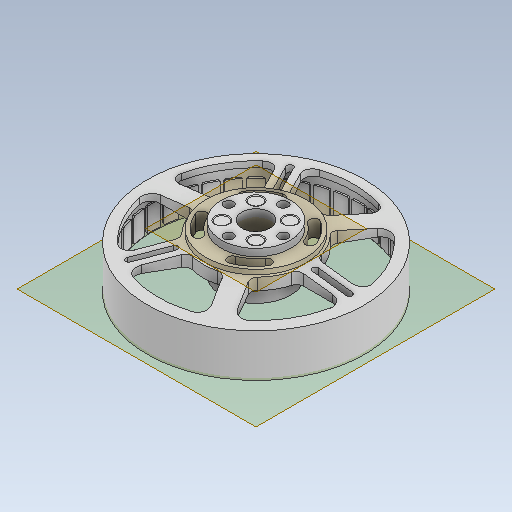
# Autodesk Inventor part: 90motor_top
Saved by Autodesk Inventor 2020 (Build 240168000, 168)
## iProperties
Created: 2020-03-23
Part Number: 90motor_top
Material: Generic
Document SubType Name: Modeling
Designer: psrobotics
Density: 1 g/cm^3
Appearance: Default
Author: psrobotics
Autodesk Inventor part; units mm, degrees
ref_plane "YZ Plane" through (0, 0, 0) normal (1, 0, 0) x (0, 1, 0)
ref_plane "XZ Plane" through (0, 0, 0) normal (0, 1, 0) x (-1, 0, 0)
ref_plane "XY Plane" through (0, 0, 0) normal (0, 0, 1) x (1, 0, 0)
sketch "Sketch1" plane through (0, 0, 0) normal (0, 1, 0) x (-1, 0, 0)
  circle A0 centre (0, 0) radius 45.5
  circle A1 centre (0, 0) radius 43
  dimension "d0" = 91
  dimension "d1" = 2.5
  constraints: 2 centre point, 2 coincident
  measures "d0" diameter of A0
  measures "d1" radial gap between concentric circles of A0 A1
extrude "Extrusion1" add sketch "Sketch1" along normal blind 23
sketch "Sketch2" plane through (0, 23, 0) normal (0, 1, 0) x (1, 0, 0)
  circle A0 centre (0, 0) radius 45.5 projected
extrude "Extrusion2" add sketch "Sketch2" against normal blind 7
sketch "Sketch3" plane through (0, 0, 0) normal (1, 0, 0) x (0, 1, 0)
  line L0 (23, -45.5) -> (23, 45.5) projected
  line L1 (0, -45.5) -> (0, 45.5) projected
  line L2 (23, -45.5) -> (23, 45.5) projected
  line L3 (23, 0) -> (23, -21)
  line L4 (23, -21) -> (21, -21)
  line L5 (0, -45.5) -> (18, -45.5)
  line L6 (0, -45.5) -> (23, -45.5) projected
  line L7 (18, -45.5) -> (21, -21)
  line L8 (23, 0) -> (33, 0)
  point P0 (0, 0)
  dimension "d6" = 21
  dimension "d7" = 2
  dimension "d8" = 18
  dimension "d9" = 10
  constraints: 10 end point, 2 perpendicular, 2 point on line, 1 midpoint
  measures "d6" distance of L3.start L3.end
  measures "d7" distance of L3.end L4.end
  measures "d8" distance of L1.start L5.end
  measures "d9" distance of L3.start L8.end
revolve "Revolution1" cut sketch "Sketch3" angle 360 about axis through (0, 23, 0) along (0, 1, 0)
ref_plane "Work Plane1" through (0, 23, 0) normal (0, 1, 0) x (1, 0, 0)
sketch "Sketch4" plane through (0, 23, 0) normal (0, 1, 0) x (1, 0, 0)
  circle A0 centre (0, 0) radius 21 projected
  circle A1 centre (0, 0) radius 22
  circle A2 centre (0, 0) radius 21 projected
  circle A3 centre (0, 0) radius 41
  line L0 (0, 0) -> (-41, 0)
  line L1 (-22, 0) -> (-41, 0)
  line L2 (-42.5, -4) -> (-42.5, 4)
  line L3 (-42.5, 4) -> (-20.5, 4)
  line L4 (-20.5, 4) -> (-20.5, -4)
  line L5 (-20.5, -4) -> (-42.5, -4)
  line L6 (-42.5, -4) -> (-20.5, 4) construction
  line L7 (-42.5, 4) -> (-20.5, -4) construction
  line L8 (-17.7859, -38.8061) -> (-24.7141, -34.8061)
  line L9 (-24.7141, -34.8061) -> (-13.7141, -15.7535)
  line L10 (-6.7859, -19.7535) -> (-17.7859, -38.8061)
  line L11 (-13.7141, -15.7535) -> (-6.7859, -19.7535)
  line L12 (24.7141, -34.8061) -> (17.7859, -38.8061)
  line L13 (17.7859, -38.8061) -> (6.7859, -19.7535)
  line L14 (13.7141, -15.7535) -> (24.7141, -34.8061)
  line L15 (6.7859, -19.7535) -> (13.7141, -15.7535)
  line L16 (42.5, 4) -> (42.5, -4)
  line L17 (42.5, -4) -> (20.5, -4)
  line L18 (20.5, 4) -> (42.5, 4)
  line L19 (20.5, -4) -> (20.5, 4)
  line L20 (17.7859, 38.8061) -> (24.7141, 34.8061)
  line L21 (24.7141, 34.8061) -> (13.7141, 15.7535)
  line L22 (6.7859, 19.7535) -> (17.7859, 38.8061)
  line L23 (13.7141, 15.7535) -> (6.7859, 19.7535)
  line L24 (-24.7141, 34.8061) -> (-17.7859, 38.8061)
  line L25 (-17.7859, 38.8061) -> (-6.7859, 19.7535)
  line L26 (-13.7141, 15.7535) -> (-24.7141, 34.8061)
  line L27 (-6.7859, 19.7535) -> (-13.7141, 15.7535)
  point P0 (-31.5, 0)
  point P1 (-23.8663, -33.3377)
  point P2 (-14.2808, -16.735)
  point P3 (-21.6333, -4)
  point P4 (-40.8044, -4)
  point P5 (16.9381, -37.3377)
  point P6 (7.3526, -20.735)
  point P7 (-7.3526, -20.735)
  point P8 (-16.9381, -37.3377)
  point P9 (40.8044, -4)
  point P10 (21.6333, -4)
  point P11 (14.2808, -16.735)
  point P12 (23.8663, -33.3377)
  point P13 (23.8663, 33.3377)
  point P14 (14.2808, 16.735)
  point P15 (21.6333, 4)
  point P16 (40.8044, 4)
  point P17 (-16.9381, 37.3377)
  point P18 (-7.3526, 20.735)
  point P19 (7.3526, 20.735)
  point P20 (16.9381, 37.3377)
  point P21 (-14.2808, 16.735)
  point P22 (-23.8663, 33.3377)
  point P23 (-40.8044, 4)
  point P24 (-21.6333, 4)
  dimension "d12" = 44
  dimension "d13" = 82
  dimension "d14" = 8
  dimension "d15" = 22
  dimension "d18" = 360
  constraints: 56 end point, 3 midpoint, 2 coincident, 2 parallel, 2 perpendicular, 1 collinear, 1 horizontal, 1 point on line, 55 other
  measures "d14" distance of L2.start L2.end
  measures "d15" distance of L2.end L3.end
extrude "Extrusion3" cut sketch "Sketch4" against normal blind 7 contours A1 L21 A3 L18 | L17 A3 L14 A1 | A1 L25 A3 L22 | L13 A3 L10 A1 | A1 L3 A3 L26 | L9 A3 L5 A1
fillet "Fillet1" radius 4 2 edges at (-16.9381, 17.2755, 37.3377) (16.9381, 17.2755, 37.3377)
fillet "Fillet2" radius 3 2 edges at (7.3526, 18.4388, 20.735) (-7.3526, 18.4388, 20.735)
pattern_circular "Circular Pattern1" count 6 over 360 about axis through (0, 22, 0) along (0, -1, 0) of "Fillet1", "Fillet2"
sketch "Sketch5" plane through (0, 23, 0) normal (0, 1, 0) x (1, 0, 0)
  line L0 (15.4641, 18.7846) -> (21.5265, 29.285) projected
  arc A0 (40.0302, 8.8649) -> (27.6923, 30.2347) centre (0, 0) ccw projected
  line L1 (36.1248, 4) -> (24, 4) projected
  arc A1 (21.12, 6.16) -> (15.8947, 15.2105) centre (0, 0) ccw projected
  arc A2 (-40.0302, -8.8649) -> (-27.6923, -30.2347) centre (0, 0) ccw projected
  line L2 (-36.1248, -4) -> (-24, -4) projected
  arc A3 (-21.12, -6.16) -> (-15.8947, -15.2105) centre (0, 0) ccw projected
  line L3 (-15.4641, -18.7846) -> (-21.5265, -29.285) projected
  arc A4 (12.3379, 39.0996) -> (-12.3379, 39.0996) centre (0, 0) ccw projected
  line L4 (14.5983, 33.285) -> (8.5359, 22.7846) projected
  arc A5 (5.2253, 21.3705) -> (-5.2253, 21.3705) centre (0, 0) ccw projected
  line L5 (-8.5359, 22.7846) -> (-14.5983, 33.285) projected
  line L6 (21.5265, -29.285) -> (15.4641, -18.7846) projected
  arc A6 (15.8947, -15.2105) -> (21.12, -6.16) centre (0, 0) ccw projected
  line L7 (24, -4) -> (36.1248, -4) projected
  arc A7 (27.6923, -30.2347) -> (40.0302, -8.8649) centre (0, 0) ccw projected
  line L8 (-14.5983, -33.285) -> (-8.5359, -22.7846) projected
  arc A8 (-5.2253, -21.3705) -> (5.2253, -21.3705) centre (0, 0) ccw projected
  line L9 (8.5359, -22.7846) -> (14.5983, -33.285) projected
  arc A9 (-12.3379, -39.0996) -> (12.3379, -39.0996) centre (0, 0) ccw projected
  arc A10 (-15.8947, 15.2105) -> (-21.12, 6.16) centre (0, 0) ccw projected
  line L10 (-24, 4) -> (-36.1248, 4) projected
  arc A11 (-27.6923, 30.2347) -> (-40.0302, 8.8649) centre (0, 0) ccw projected
  line L11 (-21.5265, 29.285) -> (-15.4641, 18.7846) projected
  circle A12 centre (0, 0) radius 45.5 projected
  circle A13 centre (0, 0) radius 21 projected
  line L12 (0, 0) -> (-22.75, -39.4042)
  line L13 (-10.5, -18.1865) -> (-21.5, -37.2391)
  line L14 (-19.5, -33.775) -> (-12.5, -21.6506) construction
  line L15 (-18.4175, -34.4) -> (-11.4175, -22.2756)
  line L16 (-13.5825, -21.0256) -> (-20.5825, -33.15)
  arc A14 (-20.5825, -33.15) -> (-18.4175, -34.4) centre (-19.5, -33.775) ccw
  arc A15 (-11.4175, -22.2756) -> (-13.5825, -21.0256) centre (-12.5, -21.6506) ccw
  point P0 (-16, -27.7128)
  dimension "d27" = 22
  dimension "d28" = 7
  dimension "d29" = 2.5
  constraints: 12 end point, 4 point on circle, 4 tangent, 3 point on line, 2 centre point, 2 midpoint, 2 parallel, 28 other
  measures "d27" distance of L13.start L13.end
  measures "d28" distance of point (-16, -27.713) L14.end
  measures "d29" diameter of A15
extrude "Extrusion4" cut sketch "Sketch5" against normal blind 7 contours A15 L15 A14 L12 | L12 A14 L16 A15
pattern_circular "Circular Pattern2" count 3 over 360 about axis through (0, 23, 0) along (0, -1, 0) of "Extrusion4"
sketch "Sketch6" plane through (0, 23, 0) normal (0, 1, 0) x (1, 0, 0)
  circle A0 centre (0, 0) radius 21 projected
  circle A1 centre (0, 0) radius 14.5
  dimension "d35" = 29
  constraints: 1 centre point, 1 coincident
  measures "d35" diameter of A1
extrude "Extrusion5" add sketch "Sketch6" along normal blind 3 contours A1
sketch "Sketch7" plane through (0, 26, 0) normal (0, 1, 0) x (1, 0, 0)
  circle A0 centre (0, 0) radius 14.5 projected
  line L0 (0, 0) -> (0, -11.45)
  circle A1 centre (0, -11.45) radius 2
  dimension "d38" = 11.45
  dimension "d39" = 4
  constraints: 2 end point, 1 centre point, 1 coincident, 1 vertical
  measures "d38" distance of L0.start L0.end
  measures "d39" diameter of A1
extrude "Extrusion6" cut sketch "Sketch7" against normal blind 20 contours A1
pattern_circular "Circular Pattern3" count 4 over 360 about axis through (0, 23, 0) along (0, 1, 0) of "Extrusion6"
sketch "Sketch8" plane through (0, 26, 0) normal (0, 1, 0) x (1, 0, 0)
  circle A0 centre (0, 0) radius 5.9
  dimension "d45" = 11.8
  constraints: 1 centre point, 1 coincident
  measures "d45" diameter of A0
extrude "Extrusion7" cut sketch "Sketch8" against normal blind 20
sketch "Sketch9" plane through (0, 16, 0) normal (0, -1, 0) x (1, 0, 0)
  circle A0 centre (0, 0) radius 14.5 projected
  circle A1 centre (0, 0) radius 5.9 projected
  circle A2 centre (-11.45, 0) radius 2 projected
  circle A3 centre (0, -11.45) radius 2 projected
  circle A4 centre (11.45, 0) radius 2 projected
  circle A5 centre (0, 11.45) radius 2 projected
  arc A6 (25, 1.25) -> (25, -1.25) centre (25, 0) ccw projected
  line L0 (25, 1.25) -> (39, 1.25) projected
  arc A7 (39, -1.25) -> (39, 1.25) centre (39, 0) ccw projected
  line L1 (39, -1.25) -> (25, -1.25) projected
  arc A8 (-11.4175, -22.2756) -> (-13.5825, -21.0256) centre (-12.5, -21.6506) ccw projected
  line L2 (-11.4175, -22.2756) -> (-18.4175, -34.4) projected
  arc A9 (-20.5825, -33.15) -> (-18.4175, -34.4) centre (-19.5, -33.775) ccw projected
  line L3 (-20.5825, -33.15) -> (-13.5825, -21.0256) projected
  arc A10 (-13.5825, 21.0256) -> (-11.4175, 22.2756) centre (-12.5, 21.6506) ccw projected
  line L4 (-13.5825, 21.0256) -> (-20.5825, 33.15) projected
  arc A11 (-18.4175, 34.4) -> (-20.5825, 33.15) centre (-19.5, 33.775) ccw projected
  line L5 (-18.4175, 34.4) -> (-11.4175, 22.2756) projected
  line L6 (21.5265, -29.285) -> (15.4641, -18.7846) projected
  arc A12 (15.8947, -15.2105) -> (15.4641, -18.7846) centre (18.0622, -17.2846) ccw projected
  arc A13 (15.8947, -15.2105) -> (21.12, -6.16) centre (0, 0) ccw projected
  arc A14 (24, -4) -> (21.12, -6.16) centre (24, -7) ccw projected
  line L7 (24, -4) -> (36.1248, -4) projected
  arc A15 (40.0302, -8.8649) -> (36.1248, -4) centre (36.1248, -8) ccw projected
  arc A16 (27.6923, -30.2347) -> (40.0302, -8.8649) centre (0, 0) ccw projected
  arc A17 (21.5265, -29.285) -> (27.6923, -30.2347) centre (24.9906, -27.285) ccw projected
  arc A18 (-27.6923, 30.2347) -> (-40.0302, 8.8649) centre (0, 0) ccw projected
  arc A19 (-21.5265, 29.285) -> (-27.6923, 30.2347) centre (-24.9906, 27.285) ccw projected
  line L8 (-21.5265, 29.285) -> (-15.4641, 18.7846) projected
  arc A20 (-15.8947, 15.2105) -> (-15.4641, 18.7846) centre (-18.0622, 17.2846) ccw projected
  arc A21 (-15.8947, 15.2105) -> (-21.12, 6.16) centre (0, 0) ccw projected
  arc A22 (-24, 4) -> (-21.12, 6.16) centre (-24, 7) ccw projected
  line L9 (-24, 4) -> (-36.1248, 4) projected
  arc A23 (-40.0302, 8.8649) -> (-36.1248, 4) centre (-36.1248, 8) ccw projected
  arc A24 (-12.3379, -39.0996) -> (12.3379, -39.0996) centre (0, 0) ccw projected
  arc A25 (-14.5983, -33.285) -> (-12.3379, -39.0996) centre (-11.1342, -35.285) ccw projected
  line L10 (-14.5983, -33.285) -> (-8.5359, -22.7846) projected
  arc A26 (-5.2253, -21.3705) -> (-8.5359, -22.7846) centre (-5.9378, -24.2846) ccw projected
  arc A27 (-5.2253, -21.3705) -> (5.2253, -21.3705) centre (0, 0) ccw projected
  arc A28 (8.5359, -22.7846) -> (5.2253, -21.3705) centre (5.9378, -24.2846) ccw projected
  line L11 (8.5359, -22.7846) -> (14.5983, -33.285) projected
  arc A29 (12.3379, -39.0996) -> (14.5983, -33.285) centre (11.1342, -35.285) ccw projected
  line L12 (15.4641, 18.7846) -> (21.5265, 29.285) projected
  arc A30 (27.6923, 30.2347) -> (21.5265, 29.285) centre (24.9906, 27.285) ccw projected
  arc A31 (40.0302, 8.8649) -> (27.6923, 30.2347) centre (0, 0) ccw projected
  arc A32 (36.1248, 4) -> (40.0302, 8.8649) centre (36.1248, 8) ccw projected
  line L13 (36.1248, 4) -> (24, 4) projected
  arc A33 (21.12, 6.16) -> (24, 4) centre (24, 7) ccw projected
  arc A34 (21.12, 6.16) -> (15.8947, 15.2105) centre (0, 0) ccw projected
  arc A35 (15.4641, 18.7846) -> (15.8947, 15.2105) centre (18.0622, 17.2846) ccw projected
  line L14 (-8.5359, 22.7846) -> (-14.5983, 33.285) projected
  arc A36 (-12.3379, 39.0996) -> (-14.5983, 33.285) centre (-11.1342, 35.285) ccw projected
  arc A37 (12.3379, 39.0996) -> (-12.3379, 39.0996) centre (0, 0) ccw projected
  arc A38 (14.5983, 33.285) -> (12.3379, 39.0996) centre (11.1342, 35.285) ccw projected
  line L15 (14.5983, 33.285) -> (8.5359, 22.7846) projected
  arc A39 (5.2253, 21.3705) -> (8.5359, 22.7846) centre (5.9378, 24.2846) ccw projected
  arc A40 (5.2253, 21.3705) -> (-5.2253, 21.3705) centre (0, 0) ccw projected
  arc A41 (-8.5359, 22.7846) -> (-5.2253, 21.3705) centre (-5.9378, 24.2846) ccw projected
  arc A42 (-21.12, -6.16) -> (-15.8947, -15.2105) centre (0, 0) ccw projected
  arc A43 (-15.4641, -18.7846) -> (-15.8947, -15.2105) centre (-18.0622, -17.2846) ccw projected
  line L16 (-15.4641, -18.7846) -> (-21.5265, -29.285) projected
  arc A44 (-27.6923, -30.2347) -> (-21.5265, -29.285) centre (-24.9906, -27.285) ccw projected
  arc A45 (-40.0302, -8.8649) -> (-27.6923, -30.2347) centre (0, 0) ccw projected
  arc A46 (-36.1248, -4) -> (-40.0302, -8.8649) centre (-36.1248, -8) ccw projected
  line L17 (-36.1248, -4) -> (-24, -4) projected
  arc A47 (-21.12, -6.16) -> (-24, -4) centre (-24, -7) ccw projected
  circle A48 centre (0, 0) radius 43 projected
extrude "Extrusion8" add sketch "Sketch9" along normal blind 10 contours A0
sketch "Sketch10" plane through (0, 23, 0) normal (0, 1, 0) x (1, 0, 0)
  circle A0 centre (0, 0) radius 14.5 projected
  circle A1 centre (0, 0) radius 21 projected
  circle A2 centre (0, 0) radius 19.5
  circle A3 centre (0, 0) radius 15.5
  line L0 (0, 0) -> (0, 19.5)
  line L1 (0, 0) -> (-19.5, 0)
  line L2 (0, 0) -> (-5.047, 18.8356)
  line L3 (0, 0) -> (-17.2175, 9.1547)
  point P0 (-13.6857, 7.2768)
  point P1 (-4.0117, 14.9719)
  dimension "d50" = 39
  dimension "d51" = 31
  dimension "d52" = 15
  dimension "d53" = 28
  constraints: 8 end point, 4 point on circle, 2 centre point, 2 coincident, 1 perpendicular, 1 vertical
  measures "d50" diameter of A2
  measures "d51" diameter of A3
  measures "d52" angle of L0 L2
  measures "d53" angle of L1 L3
extrude "Extrusion9" cut sketch "Sketch10" against normal blind 10 contours A3 L3 A2 L2
fillet "Fillet3" radius 2 4 edges at (-17.2175, 19.5, -9.1547) (-13.6857, 19.5, -7.2768) (-4.0117, 19.5, -14.9719) (-5.047, 19.5, -18.8356)
pattern_circular "Circular Pattern4" count 4 over 360 about axis through (0, 26, 0) along (0, -1, 0) of "Extrusion9", "Fillet3"
sketch "Sketch11" plane through (0, 26, 0) normal (0, 1, 0) x (1, 0, 0)
  circle A0 centre (0, 0) radius 5.9 projected
  circle A1 centre (-11.45, 0) radius 2 projected
  circle A2 centre (0, 11.45) radius 2 projected
  circle A3 centre (11.45, 0) radius 2 projected
  circle A4 centre (0, -11.45) radius 2 projected
  circle A5 centre (0, 0) radius 14.5 projected
  line L0 (0, 11.45) -> (11.45, 0)
  line L1 (5.725, 5.725) -> (7.1392, 7.1392)
  circle A6 centre (7.1392, 7.1392) radius 3
  dimension "d60" = 2
  dimension "d61" = 6
  constraints: 4 end point, 1 centre point, 1 coincident, 1 midpoint, 1 perpendicular
  measures "d60" distance of L1.start L1.end
  measures "d61" diameter of A6
extrude "Extrusion10" cut sketch "Sketch11" against normal blind 0.2 contours A6 L0 | L0 A6
pattern_circular "Circular Pattern5" count 4 over 360 about axis through (0, 23, 0) along (0, 1, 0) of "Extrusion10"
fillet "Fillet4" radius 0.5 4 edges at (-7.1392, 25.8, -4.1392) (4.1392, 25.8, -7.1392) (7.1392, 25.8, 4.1392) (-4.1392, 25.8, 7.1392)
thicken "Thicken1" operation add thickness 0.5 both sides no extend neighbours yes toward (-0.8829476, 0, 0.4694716) faces at (-37.9667, 10.6667, 20.1873)
ref_plane "Work Plane2" through (0, 1, 0) normal (0, -1, 0) x (1, 0, 0)
sketch "Sketch12" plane through (0, 1, 0) normal (0, -1, 0) x (1, 0, 0)
  circle A0 centre (0, 0) radius 43.5 projected
  arc A1 (-8.7932, 12.7644) -> (-14.4153, 5.6965) centre (0, 0) ccw projected
  arc A2 (-18.1353, 7.1665) -> (-14.4153, 5.6965) centre (-16.2753, 6.4315) ccw projected
  arc A3 (-11.0624, 16.0584) -> (-18.1353, 7.1665) centre (0, 0) ccw projected
  arc A4 (-8.7932, 12.7644) -> (-11.0624, 16.0584) centre (-9.9278, 14.4114) ccw projected
  arc A5 (12.7644, 8.7932) -> (5.6965, 14.4153) centre (0, 0) ccw projected
  arc A6 (7.1665, 18.1353) -> (5.6965, 14.4153) centre (6.4315, 16.2753) ccw projected
  arc A7 (16.0584, 11.0624) -> (7.1665, 18.1353) centre (0, 0) ccw projected
  arc A8 (12.7644, 8.7932) -> (16.0584, 11.0624) centre (14.4114, 9.9278) ccw projected
  arc A9 (8.7932, -12.7644) -> (14.4153, -5.6965) centre (0, 0) ccw projected
  arc A10 (18.1353, -7.1665) -> (14.4153, -5.6965) centre (16.2753, -6.4315) ccw projected
  arc A11 (11.0624, -16.0584) -> (18.1353, -7.1665) centre (0, 0) ccw projected
  arc A12 (8.7932, -12.7644) -> (11.0624, -16.0584) centre (9.9278, -14.4114) ccw projected
  arc A13 (-12.7644, -8.7932) -> (-5.6965, -14.4153) centre (0, 0) ccw projected
  arc A14 (-7.1665, -18.1353) -> (-5.6965, -14.4153) centre (-6.4315, -16.2753) ccw projected
  arc A15 (-16.0584, -11.0624) -> (-7.1665, -18.1353) centre (0, 0) ccw projected
  arc A16 (-12.7644, -8.7932) -> (-16.0584, -11.0624) centre (-14.4114, -9.9278) ccw projected
  circle A17 centre (0, 0) radius 14.5 projected
  arc A18 (25, 1.25) -> (25, -1.25) centre (25, 0) ccw projected
  line L0 (25, 1.25) -> (39, 1.25) projected
  arc A19 (39, -1.25) -> (39, 1.25) centre (39, 0) ccw projected
  line L1 (39, -1.25) -> (25, -1.25) projected
  arc A20 (-11.4175, -22.2756) -> (-13.5825, -21.0256) centre (-12.5, -21.6506) ccw projected
  line L2 (-11.4175, -22.2756) -> (-18.4175, -34.4) projected
  arc A21 (-20.5825, -33.15) -> (-18.4175, -34.4) centre (-19.5, -33.775) ccw projected
  line L3 (-20.5825, -33.15) -> (-13.5825, -21.0256) projected
  arc A22 (-13.5825, 21.0256) -> (-11.4175, 22.2756) centre (-12.5, 21.6506) ccw projected
  line L4 (-13.5825, 21.0256) -> (-20.5825, 33.15) projected
  arc A23 (-18.4175, 34.4) -> (-20.5825, 33.15) centre (-19.5, 33.775) ccw projected
  line L5 (-18.4175, 34.4) -> (-11.4175, 22.2756) projected
  line L6 (21.5265, -29.285) -> (15.4641, -18.7846) projected
  arc A24 (15.8947, -15.2105) -> (15.4641, -18.7846) centre (18.0622, -17.2846) ccw projected
  arc A25 (15.8947, -15.2105) -> (21.12, -6.16) centre (0, 0) ccw projected
  arc A26 (24, -4) -> (21.12, -6.16) centre (24, -7) ccw projected
  line L7 (24, -4) -> (36.1248, -4) projected
  arc A27 (40.0302, -8.8649) -> (36.1248, -4) centre (36.1248, -8) ccw projected
  arc A28 (27.6923, -30.2347) -> (40.0302, -8.8649) centre (0, 0) ccw projected
  arc A29 (21.5265, -29.285) -> (27.6923, -30.2347) centre (24.9906, -27.285) ccw projected
  arc A30 (-27.6923, 30.2347) -> (-40.0302, 8.8649) centre (0, 0) ccw projected
  arc A31 (-21.5265, 29.285) -> (-27.6923, 30.2347) centre (-24.9906, 27.285) ccw projected
  line L8 (-21.5265, 29.285) -> (-15.4641, 18.7846) projected
  arc A32 (-15.8947, 15.2105) -> (-15.4641, 18.7846) centre (-18.0622, 17.2846) ccw projected
  arc A33 (-15.8947, 15.2105) -> (-21.12, 6.16) centre (0, 0) ccw projected
  arc A34 (-24, 4) -> (-21.12, 6.16) centre (-24, 7) ccw projected
  line L9 (-24, 4) -> (-36.1248, 4) projected
  arc A35 (-40.0302, 8.8649) -> (-36.1248, 4) centre (-36.1248, 8) ccw projected
  arc A36 (-12.3379, -39.0996) -> (12.3379, -39.0996) centre (0, 0) ccw projected
  arc A37 (-14.5983, -33.285) -> (-12.3379, -39.0996) centre (-11.1342, -35.285) ccw projected
  line L10 (-14.5983, -33.285) -> (-8.5359, -22.7846) projected
  arc A38 (-5.2253, -21.3705) -> (-8.5359, -22.7846) centre (-5.9378, -24.2846) ccw projected
  arc A39 (-5.2253, -21.3705) -> (5.2253, -21.3705) centre (0, 0) ccw projected
  arc A40 (8.5359, -22.7846) -> (5.2253, -21.3705) centre (5.9378, -24.2846) ccw projected
  line L11 (8.5359, -22.7846) -> (14.5983, -33.285) projected
  arc A41 (12.3379, -39.0996) -> (14.5983, -33.285) centre (11.1342, -35.285) ccw projected
  line L12 (15.4641, 18.7846) -> (21.5265, 29.285) projected
  arc A42 (27.6923, 30.2347) -> (21.5265, 29.285) centre (24.9906, 27.285) ccw projected
  arc A43 (40.0302, 8.8649) -> (27.6923, 30.2347) centre (0, 0) ccw projected
  arc A44 (36.1248, 4) -> (40.0302, 8.8649) centre (36.1248, 8) ccw projected
  line L13 (36.1248, 4) -> (24, 4) projected
  arc A45 (21.12, 6.16) -> (24, 4) centre (24, 7) ccw projected
  arc A46 (21.12, 6.16) -> (15.8947, 15.2105) centre (0, 0) ccw projected
  arc A47 (15.4641, 18.7846) -> (15.8947, 15.2105) centre (18.0622, 17.2846) ccw projected
  line L14 (-8.5359, 22.7846) -> (-14.5983, 33.285) projected
  arc A48 (-12.3379, 39.0996) -> (-14.5983, 33.285) centre (-11.1342, 35.285) ccw projected
  arc A49 (12.3379, 39.0996) -> (-12.3379, 39.0996) centre (0, 0) ccw projected
  arc A50 (14.5983, 33.285) -> (12.3379, 39.0996) centre (11.1342, 35.285) ccw projected
  line L15 (14.5983, 33.285) -> (8.5359, 22.7846) projected
  arc A51 (5.2253, 21.3705) -> (8.5359, 22.7846) centre (5.9378, 24.2846) ccw projected
  arc A52 (5.2253, 21.3705) -> (-5.2253, 21.3705) centre (0, 0) ccw projected
  arc A53 (-8.5359, 22.7846) -> (-5.2253, 21.3705) centre (-5.9378, 24.2846) ccw projected
  arc A54 (-21.12, -6.16) -> (-15.8947, -15.2105) centre (0, 0) ccw projected
  arc A55 (-15.4641, -18.7846) -> (-15.8947, -15.2105) centre (-18.0622, -17.2846) ccw projected
  line L16 (-15.4641, -18.7846) -> (-21.5265, -29.285) projected
  arc A56 (-27.6923, -30.2347) -> (-21.5265, -29.285) centre (-24.9906, -27.285) ccw projected
  arc A57 (-40.0302, -8.8649) -> (-27.6923, -30.2347) centre (0, 0) ccw projected
  arc A58 (-36.1248, -4) -> (-40.0302, -8.8649) centre (-36.1248, -8) ccw projected
  line L17 (-36.1248, -4) -> (-24, -4) projected
  arc A59 (-21.12, -6.16) -> (-24, -4) centre (-24, -7) ccw projected
  circle A60 centre (0, 0) radius 43.5 projected
  circle A61 centre (0, 0) radius 42.8
  line L18 (-45, -2.75) -> (-45, 2.75)
  line L19 (-45, 2.75) -> (-42, 2.75)
  line L20 (-42, 2.75) -> (-42, -2.75)
  line L21 (-42, -2.75) -> (-45, -2.75)
  circle A62 centre (0, 0) radius 43.5 projected
  line L22 (-45, -2.75) -> (-42, 2.75) construction
  line L23 (-45, 2.75) -> (-42, -2.75) construction
  line L24 (-43.5, 0) -> (0, 0)
  point P0 (-43.413, -2.75)
  point P1 (-42.7116, -2.75)
  point P2 (-42.7116, 2.75)
  point P3 (-43.413, 2.75)
  dimension "d71" = 0.7
  dimension "d72" = 5.5
  dimension "d73" = 3
  constraints: 14 end point, 2 midpoint, 2 parallel, 2 perpendicular, 1 centre point, 1 coincident, 1 horizontal, 1 horizontal alignment, 1 other
  measures "d71" radial gap between concentric circles of A60 A61
  measures "d72" distance of L18.start L18.end
  measures "d73" distance of L18.end L19.end
extrude "Extrusion11" add sketch "Sketch12" against normal blind 10 contours L19 A61 L24 A0 | A0 L24 A61 L21
fillet "Fillet5" radius 0.5 4 edges at (-43.0623, 1, 2.75) (-43.0623, 1, -2.75) (-43.0623, 11, -2.75) (-43.0623, 11, 2.75)
pattern_circular "Circular Pattern6" count 40 over 360 about axis through (0, 0, 0) along (0, 1, 0) of "Extrusion11", "Fillet5"
body "Solid1"
